Autodesk Fusion 360 part; units mm, degrees
(part 2 of 8)
  spline S29 degree 5 poles (575.857, 282.4121) (575.8643, 282.439) (575.8953, 282.5546) (575.9497, 282.7591) (576.0262, 283.0527) (576.1235, 283.4362) (576.2331, 283.8827) (576.3395, 284.3305) (576.4425, 284.7793) (576.5422, 285.2294) (576.6386, 285.6806) (576.7319, 286.1328) (576.8222, 286.5861) (576.9096, 287.0403) (576.9942, 287.4954) (577.0761, 287.9513) (577.1553, 288.4081) (577.2319, 288.8657) (577.3058, 289.3241) (577.3772, 289.7833) (577.446, 290.2433) (577.5123, 290.704) (577.5762, 291.1654) (577.6376, 291.6276) (577.6967, 292.0904) (577.7535, 292.5539) (577.8079, 293.018) (577.8601, 293.4828) (577.91, 293.9481) (577.9577, 294.4141) (578.0032, 294.8806) (578.0465, 295.3478) (578.0876, 295.8155) (578.1266, 296.2837) (578.1635, 296.7525) (578.1984, 297.2218) (578.2311, 297.6916) (578.2618, 298.1619) (578.2905, 298.6327) (578.3171, 299.1039) (578.3418, 299.5757) (578.3645, 300.0479) (578.3852, 300.5205) (578.404, 300.9936) (578.4208, 301.4672) (578.4358, 301.9411) (578.4488, 302.4154) (578.4599, 302.8902) (578.4692, 303.3654) (578.4766, 303.8409) (578.4822, 304.3168) (578.4859, 304.7931) (578.4878, 305.2698) (578.4879, 305.7468) (578.4862, 306.2242) (578.4827, 306.7019) (578.4775, 307.1799) (578.4704, 307.6583) (578.4617, 308.137) (578.4511, 308.616) (578.4389, 309.0953) (578.4249, 309.5749) (578.4123, 309.9589) (578.4021, 310.2469) (578.395, 310.4391) (578.3913, 310.5351) knots 0.13851185 0.13851185 0.13851185 0.13851185 0.13851185 0.13851185 0.14285714 0.15714286 0.17142857 0.18571429 0.2 0.21428571 0.22857143 0.24285714 0.25714286 0.27142857 0.28571429 0.3 0.31428571 0.32857143 0.34285714 0.35714286 0.37142857 0.38571429 0.4 0.41428571 0.42857143 0.44285714 0.45714286 0.47142857 0.48571429 0.5 0.51428571 0.52857143 0.54285714 0.55714286 0.57142857 0.58571429 0.6 0.61428571 0.62857143 0.64285714 0.65714286 0.67142857 0.68571429 0.7 0.71428571 0.72857143 0.74285714 0.75714286 0.77142857 0.78571429 0.8 0.81428571 0.82857143 0.84285714 0.85714286 0.87142857 0.88571429 0.9 0.91428571 0.92857143 0.94285714 0.95714286 0.97142857 0.98571429 1 1 1 1 1 1
  arc A15 (578.3913, 310.5351) -> (569.3228, 314.2914) centre (452.3696, 19.1166) ccw
  spline S30 degree 5 poles (569.3228, 314.2914) (569.2522, 314.2261) (569.1113, 314.0953) (568.9004, 313.8988) (568.62, 313.6362) (568.271, 313.307) (567.9234, 312.9767) (567.5773, 312.6455) (567.2326, 312.3132) (566.8893, 311.9799) (566.5476, 311.6456) (566.2073, 311.3103) (565.8686, 310.9739) (565.5313, 310.6365) (565.1956, 310.2982) (564.8615, 309.9587) (564.5289, 309.6183) (564.1979, 309.2768) (563.8684, 308.9342) (563.5406, 308.5906) (563.2144, 308.246) (562.8898, 307.9003) (562.5669, 307.5536) (562.2457, 307.2058) (561.9261, 306.8569) (561.6083, 306.5069) (561.2921, 306.1559) (560.9777, 305.8038) (560.6651, 305.4507) (560.3543, 305.0964) (560.0452, 304.741) (559.738, 304.3846) (559.4326, 304.027) (559.1291, 303.6683) (558.8275, 303.3085) (558.5278, 302.9476) (558.23, 302.5855) (557.9343, 302.2223) (557.6405, 301.858) (557.3488, 301.4925) (557.0591, 301.1258) (556.7715, 300.7579) (556.486, 300.3889) (556.2027, 300.0186) (555.9216, 299.6472) (555.6427, 299.2745) (555.3661, 298.9006) (555.0918, 298.5254) (554.82, 298.149) (554.5506, 297.7713) (554.2836, 297.3922) (554.0191, 297.0119) (553.7571, 296.6303) (553.4978, 296.2474) (553.2411, 295.863) (552.9873, 295.4773) (552.7364, 295.0901) (552.4887, 294.7013) (552.2441, 294.3111) (552.0027, 293.9193) (551.7645, 293.526) (551.5621, 293.1861) (551.4086, 292.9243) (551.3024, 292.7413) (551.2427, 292.6376) (551.2287, 292.6134) knots -1 -1 -1 -1 -1 -1 -0.98571429 -0.97142857 -0.95714286 -0.94285714 -0.92857143 -0.91428571 -0.9 -0.88571429 -0.87142857 -0.85714286 -0.84285714 -0.82857143 -0.81428571 -0.8 -0.78571429 -0.77142857 -0.75714286 -0.74285714 -0.72857143 -0.71428571 -0.7 -0.68571429 -0.67142857 -0.65714286 -0.64285714 -0.62857143 -0.61428571 -0.6 -0.58571429 -0.57142857 -0.55714286 -0.54285714 -0.52857143 -0.51428571 -0.5 -0.48571429 -0.47142857 -0.45714286 -0.44285714 -0.42857143 -0.41428571 -0.4 -0.38571429 -0.37142857 -0.35714286 -0.34285714 -0.32857143 -0.31428571 -0.3 -0.28571429 -0.27142857 -0.25714286 -0.24285714 -0.22857143 -0.21428571 -0.2 -0.18571429 -0.17142857 -0.15714286 -0.14285714 -0.13851185 -0.13851185 -0.13851185 -0.13851185 -0.13851185 -0.13851185
  spline S31 degree 3 poles (549.3212, 291.9095) (549.516, 291.8402) (549.7224, 291.8097) (550.1354, 291.8295) (550.338, 291.8797) (550.672, 292.0358) (550.8074, 292.1265) (551.0461, 292.3458) (551.1479, 292.473) (551.2287, 292.6134) knots 0 0 0 0 0.062015 0.062015 0.12403 0.12403 0.172638 0.172638 0.221247 0.221247 0.221247 0.221247
  arc A16 (549.3212, 291.9095) -> (541.5184, 294.5582) centre (452.3696, 19.1166) ccw
  spline S32 degree 3 poles (540.4336, 296.2779) (540.4064, 296.073) (540.4194, 295.8647) (540.5245, 295.4649) (540.6156, 295.2771) (540.8378, 294.9828) (540.9546, 294.8692) (541.2186, 294.6813) (541.3643, 294.6081) (541.5184, 294.5582) knots 0 0 0 0 0.062015 0.062015 0.12403 0.12403 0.172638 0.172638 0.221247 0.221247 0.221247 0.221247
  spline S33 degree 5 poles (540.4336, 296.2779) (540.4373, 296.3055) (540.453, 296.4242) (540.4802, 296.634) (540.5177, 296.9352) (540.5641, 297.328) (540.6146, 297.7851) (540.6615, 298.2428) (540.7051, 298.7013) (540.7452, 299.1606) (540.7819, 299.6205) (540.8153, 300.081) (540.8457, 300.5422) (540.873, 301.0039) (540.8975, 301.4661) (540.9192, 301.9288) (540.9381, 302.3921) (540.9543, 302.8557) (540.9678, 303.3199) (540.9786, 303.7845) (540.9868, 304.2495) (540.9924, 304.7149) (540.9955, 305.1808) (540.9961, 305.647) (540.9943, 306.1136) (540.9901, 306.5805) (540.9835, 307.0477) (540.9745, 307.5153) (540.9633, 307.9832) (540.9497, 308.4514) (540.9339, 308.9199) (540.9159, 309.3887) (540.8956, 309.8578) (540.8732, 310.3271) (540.8486, 310.7967) (540.8219, 311.2665) (540.793, 311.7366) (540.7621, 312.2068) (540.729, 312.6773) (540.694, 313.1481) (540.6568, 313.619) (540.6177, 314.0901) (540.5765, 314.5614) (540.5334, 315.0329) (540.4883, 315.5046) (540.4412, 315.9764) (540.3923, 316.4484) (540.3413, 316.9206) (540.2885, 317.3929) (540.2338, 317.8653) (540.1772, 318.3379) (540.1187, 318.8106) (540.0584, 319.2834) (539.9962, 319.7564) (539.9322, 320.2295) (539.8664, 320.7026) (539.7988, 321.1759) (539.7294, 321.6493) (539.6582, 322.1227) (539.5852, 322.5962) (539.5105, 323.0698) (539.434, 323.5435) (539.3715, 323.9225) (539.3237, 324.2068) (539.2916, 324.3964) (539.2754, 324.4911) knots 0.13851185 0.13851185 0.13851185 0.13851185 0.13851185 0.13851185 0.14285714 0.15714286 0.17142857 0.18571429 0.2 0.21428571 0.22857143 0.24285714 0.25714286 0.27142857 0.28571429 0.3 0.31428571 0.32857143 0.34285714 0.35714286 0.37142857 0.38571429 0.4 0.41428571 0.42857143 0.44285714 0.45714286 0.47142857 0.48571429 0.5 0.51428571 0.52857143 0.54285714 0.55714286 0.57142857 0.58571429 0.6 0.61428571 0.62857143 0.64285714 0.65714286 0.67142857 0.68571429 0.7 0.71428571 0.72857143 0.74285714 0.75714286 0.77142857 0.78571429 0.8 0.81428571 0.82857143 0.84285714 0.85714286 0.87142857 0.88571429 0.9 0.91428571 0.92857143 0.94285714 0.95714286 0.97142857 0.98571429 1 1 1 1 1 1
  arc A17 (539.2754, 324.4911) -> (529.7942, 327.0316) centre (452.3696, 19.1166) ccw
  spline S34 degree 5 poles (529.7942, 327.0316) (529.7328, 326.9576) (529.6101, 326.8096) (529.4267, 326.5872) (529.183, 326.2903) (528.8799, 325.9183) (528.5784, 325.5455) (528.2784, 325.1719) (527.9801, 324.7975) (527.6833, 324.4222) (527.3881, 324.0462) (527.0945, 323.6693) (526.8025, 323.2916) (526.5122, 322.9131) (526.2236, 322.5338) (525.9366, 322.1537) (525.6513, 321.7727) (525.3677, 321.3909) (525.0858, 321.0083) (524.8056, 320.6249) (524.5272, 320.2406) (524.2505, 319.8555) (523.9756, 319.4696) (523.7025, 319.0828) (523.4312, 318.6952) (523.1617, 318.3068) (522.8941, 317.9175) (522.6284, 317.5274) (522.3645, 317.1364) (522.1026, 316.7446) (521.8426, 316.352) (521.5845, 315.9585) (521.3284, 315.5641) (521.0743, 315.1689) (520.8222, 314.7728) (520.5722, 314.3758) (520.3243, 313.978) (520.0784, 313.5793) (519.8347, 313.1797) (519.5932, 312.7792) (519.3539, 312.3779) (519.1168, 311.9756) (518.8819, 311.5725) (518.6493, 311.1684) (518.4191, 310.7635) (518.1912, 310.3576) (517.9658, 309.9508) (517.7429, 309.543) (517.5225, 309.1343) (517.3047, 308.7246) (517.0894, 308.314) (516.8768, 307.9024) (516.6669, 307.4899) (516.4598, 307.0763) (516.2555, 306.6618) (516.0542, 306.2462) (515.856, 305.8296) (515.6611, 305.4118) (515.4696, 304.993) (515.2814, 304.5731) (515.0965, 304.152) (514.9403, 303.7886) (514.8222, 303.509) (514.7409, 303.3138) (514.6951, 303.2031) (514.6845, 303.1773) knots -1 -1 -1 -1 -1 -1 -0.98571429 -0.97142857 -0.95714286 -0.94285714 -0.92857143 -0.91428571 -0.9 -0.88571429 -0.87142857 -0.85714286 -0.84285714 -0.82857143 -0.81428571 -0.8 -0.78571429 -0.77142857 -0.75714286 -0.74285714 -0.72857143 -0.71428571 -0.7 -0.68571429 -0.67142857 -0.65714286 -0.64285714 -0.62857143 -0.61428571 -0.6 -0.58571429 -0.57142857 -0.55714286 -0.54285714 -0.52857143 -0.51428571 -0.5 -0.48571429 -0.47142857 -0.45714286 -0.44285714 -0.42857143 -0.41428571 -0.4 -0.38571429 -0.37142857 -0.35714286 -0.34285714 -0.32857143 -0.31428571 -0.3 -0.28571429 -0.27142857 -0.25714286 -0.24285714 -0.22857143 -0.21428571 -0.2 -0.18571429 -0.17142857 -0.15714286 -0.14285714 -0.13851185 -0.13851185 -0.13851185 -0.13851185 -0.13851185 -0.13851185
  spline S35 degree 3 poles (512.8852, 302.2304) (513.0873, 302.1872) (513.296, 302.1839) (513.7028, 302.2574) (513.8971, 302.3336) (514.2079, 302.532) (514.3303, 302.6396) (514.5383, 302.8881) (514.6227, 303.0276) (514.6845, 303.1773) knots 0 0 0 0 0.062015 0.062015 0.12403 0.12403 0.172638 0.172638 0.221247 0.221247 0.221247 0.221247
  arc A18 (512.8852, 302.2304) -> (504.8034, 303.838) centre (452.3696, 19.1166) ccw
  spline S36 degree 3 poles (503.5034, 305.4014) (503.5031, 305.1947) (503.5432, 304.9899) (503.6997, 304.6072) (503.8145, 304.4329) (504.0732, 304.1701) (504.2038, 304.0727) (504.4901, 303.9209) (504.644, 303.8673) (504.8034, 303.838) knots 0 0 0 0 0.062015 0.062015 0.12403 0.12403 0.172638 0.172638 0.221247 0.221247 0.221247 0.221247
  spline S37 degree 5 poles (503.5034, 305.4014) (503.5034, 305.4293) (503.5035, 305.549) (503.5031, 305.7606) (503.501, 306.064) (503.4957, 306.4596) (503.4861, 306.9193) (503.4729, 307.3793) (503.4562, 307.8395) (503.436, 308.3001) (503.4124, 308.7608) (503.3854, 309.2218) (503.3553, 309.683) (503.3222, 310.1443) (503.2861, 310.6058) (503.2472, 311.0674) (503.2055, 311.5291) (503.1611, 311.991) (503.1139, 312.4529) (503.0639, 312.9149) (503.0114, 313.377) (502.9562, 313.8392) (502.8984, 314.3015) (502.8382, 314.7638) (502.7755, 315.2261) (502.7103, 315.6885) (502.6428, 316.1509) (502.5729, 316.6133) (502.5007, 317.0757) (502.4262, 317.5382) (502.3493, 318.0006) (502.2703, 318.463) (502.1889, 318.9254) (502.1054, 319.3878) (502.0198, 319.8501) (501.9319, 320.3125) (501.842, 320.7747) (501.7499, 321.2369) (501.6557, 321.6991) (501.5595, 322.1612) (501.4612, 322.6233) (501.3609, 323.0853) (501.2586, 323.5472) (501.1543, 324.009) (501.048, 324.4708) (500.9398, 324.9324) (500.8296, 325.394) (500.7175, 325.8555) (500.6035, 326.3168) (500.4876, 326.7781) (500.3698, 327.2392) (500.2501, 327.7003) (500.1286, 328.1612) (500.0052, 328.622) (499.88, 329.0826) (499.753, 329.5431) (499.6242, 330.0035) (499.4936, 330.4638) (499.3612, 330.9239) (499.227, 331.3839) (499.0912, 331.8437) (498.9535, 332.3033) (498.842, 332.6709) (498.7576, 332.9465) (498.7009, 333.1303) (498.6725, 333.2221) knots 0.13851185 0.13851185 0.13851185 0.13851185 0.13851185 0.13851185 0.14285714 0.15714286 0.17142857 0.18571429 0.2 0.21428571 0.22857143 0.24285714 0.25714286 0.27142857 0.28571429 0.3 0.31428571 0.32857143 0.34285714 0.35714286 0.37142857 0.38571429 0.4 0.41428571 0.42857143 0.44285714 0.45714286 0.47142857 0.48571429 0.5 0.51428571 0.52857143 0.54285714 0.55714286 0.57142857 0.58571429 0.6 0.61428571 0.62857143 0.64285714 0.65714286 0.67142857 0.68571429 0.7 0.71428571 0.72857143 0.74285714 0.75714286 0.77142857 0.78571429 0.8 0.81428571 0.82857143 0.84285714 0.85714286 0.87142857 0.88571429 0.9 0.91428571 0.92857143 0.94285714 0.95714286 0.97142857 0.98571429 1 1 1 1 1 1
  arc A19 (498.6725, 333.2221) -> (488.9408, 334.5033) centre (452.3696, 19.1166) ccw
  spline S38 degree 5 poles (488.9408, 334.5033) (488.8896, 334.422) (488.7873, 334.2591) (488.6345, 334.0148) (488.4316, 333.6885) (488.1797, 333.2802) (487.9294, 332.8712) (487.6808, 332.4617) (487.4338, 332.0515) (487.1886, 331.6407) (486.945, 331.2294) (486.7031, 330.8174) (486.4629, 330.4048) (486.2245, 329.9917) (485.9878, 329.5779) (485.7529, 329.1636) (485.5198, 328.7486) (485.2884, 328.3331) (485.0589, 327.9169) (484.8312, 327.5002) (484.6053, 327.0829) (484.3812, 326.665) (484.1591, 326.2465) (483.9388, 325.8274) (483.7204, 325.4077) (483.5039, 324.9874) (483.2894, 324.5665) (483.0769, 324.1451) (482.8663, 323.723) (482.6577, 323.3004) (482.4512, 322.8771) (482.2467, 322.4533) (482.0443, 322.0289) (481.8439, 321.6039) (481.6457, 321.1783) (481.4497, 320.7521) (481.2558, 320.3253) (481.0641, 319.8979) (480.8746, 319.4699) (480.6874, 319.0414) (480.5025, 318.6122) (480.3199, 318.1824) (480.1397, 317.7521) (479.9619, 317.3211) (479.7864, 316.8896) (479.6135, 316.4574) (479.4431, 316.0247) (479.2753, 315.5913) (479.1102, 315.1573) (478.9477, 314.7227) (478.7879, 314.2875) (478.6309, 313.8517) (478.4766, 313.4153) (478.3252, 312.9783) (478.1767, 312.5406) (478.0314, 312.1023) (477.8893, 311.6634) (477.7506, 311.2238) (477.6154, 310.7835) (477.4836, 310.3426) (477.3553, 309.901) (477.2478, 309.5203) (477.1673, 309.2277) (477.1121, 309.0235) (477.0812, 308.9079) (477.074, 308.8809) knots -1 -1 -1 -1 -1 -1 -0.98571429 -0.97142857 -0.95714286 -0.94285714 -0.92857143 -0.91428571 -0.9 -0.88571429 -0.87142857 -0.85714286 -0.84285714 -0.82857143 -0.81428571 -0.8 -0.78571429 -0.77142857 -0.75714286 -0.74285714 -0.72857143 -0.71428571 -0.7 -0.68571429 -0.67142857 -0.65714286 -0.64285714 -0.62857143 -0.61428571 -0.6 -0.58571429 -0.57142857 -0.55714286 -0.54285714 -0.52857143 -0.51428571 -0.5 -0.48571429 -0.47142857 -0.45714286 -0.44285714 -0.42857143 -0.41428571 -0.4 -0.38571429 -0.37142857 -0.35714286 -0.34285714 -0.32857143 -0.31428571 -0.3 -0.28571429 -0.27142857 -0.25714286 -0.24285714 -0.22857143 -0.21428571 -0.2 -0.18571429 -0.17142857 -0.15714286 -0.14285714 -0.13851185 -0.13851185 -0.13851185 -0.13851185 -0.13851185 -0.13851185
  spline S39 degree 3 poles (475.4137, 307.7072) (475.6197, 307.6908) (475.827, 307.7147) (476.2208, 307.8407) (476.4035, 307.9416) (476.6857, 308.1789) (476.793, 308.3015) (476.9668, 308.5751) (477.0323, 308.7243) (477.074, 308.8809) knots 0 0 0 0 0.062015 0.062015 0.12403 0.12403 0.172638 0.172638 0.221247 0.221247 0.221247 0.221247
  arc A20 (475.4137, 307.7072) -> (467.1912, 308.2461) centre (452.3696, 19.1166) ccw
  spline S40 degree 3 poles (465.6983, 309.6265) (465.725, 309.4215) (465.7915, 309.2237) (465.9965, 308.8647) (466.1331, 308.7069) (466.4239, 308.4802) (466.5662, 308.4006) (466.8698, 308.2875) (467.0294, 308.2544) (467.1912, 308.2461) knots 0 0 0 0 0.062015 0.062015 0.12403 0.12403 0.172638 0.172638 0.221247 0.221247 0.221247 0.221247
  spline S41 degree 5 poles (465.6983, 309.6265) (465.6947, 309.6542) (465.6791, 309.7729) (465.6511, 309.9825) (465.6094, 310.2831) (465.5526, 310.6746) (465.483, 311.1291) (465.4099, 311.5835) (465.3333, 312.0376) (465.2531, 312.4916) (465.1695, 312.9453) (465.0827, 313.3988) (464.9926, 313.8521) (464.8996, 314.3052) (464.8036, 314.758) (464.7048, 315.2106) (464.6031, 315.6629) (464.4988, 316.115) (464.3917, 316.5668) (464.2819, 317.0184) (464.1694, 317.4697) (464.0544, 317.9207) (463.9368, 318.3715) (463.8167, 318.8219) (463.6942, 319.2721) (463.5693, 319.7221) (463.442, 320.1717) (463.3123, 320.621) (463.1803, 321.0701) (463.0461, 321.5188) (462.9096, 321.9673) (462.7708, 322.4154) (462.6298, 322.8632) (462.4867, 323.3108) (462.3414, 323.758) (462.194, 324.2049) (462.0444, 324.6514) (461.8928, 325.0977) (461.7391, 325.5436) (461.5834, 325.9892) (461.4257, 326.4345) (461.2659, 326.8794) (461.1042, 327.324) (460.9405, 327.7683) (460.7749, 328.2122) (460.6073, 328.6558) (460.4378, 329.099) (460.2664, 329.5419) (460.0932, 329.9845) (459.918, 330.4266) (459.741, 330.8685) (459.5622, 331.3099) (459.3816, 331.751) (459.1991, 332.1918) (459.0149, 332.6322) (458.8288, 333.0722) (458.641, 333.5118) (458.4515, 333.9511) (458.2601, 334.39) (458.0671, 334.8285) (457.8724, 335.2666) (457.6759, 335.7044) (457.5174, 336.0543) (457.3977, 336.3165) (457.3176, 336.4913) (457.2774, 336.5787) knots 0.13851185 0.13851185 0.13851185 0.13851185 0.13851185 0.13851185 0.14285714 0.15714286 0.17142857 0.18571429 0.2 0.21428571 0.22857143 0.24285714 0.25714286 0.27142857 0.28571429 0.3 0.31428571 0.32857143 0.34285714 0.35714286 0.37142857 0.38571429 0.4 0.41428571 0.42857143 0.44285714 0.45714286 0.47142857 0.48571429 0.5 0.51428571 0.52857143 0.54285714 0.55714286 0.57142857 0.58571429 0.6 0.61428571 0.62857143 0.64285714 0.65714286 0.67142857 0.68571429 0.7 0.71428571 0.72857143 0.74285714 0.75714286 0.77142857 0.78571429 0.8 0.81428571 0.82857143 0.84285714 0.85714286 0.87142857 0.88571429 0.9 0.91428571 0.92857143 0.94285714 0.95714286 0.97142857 0.98571429 1 1 1 1 1 1
  arc A21 (457.2774, 336.5787) -> (447.4617, 336.5787) centre (452.3696, 19.1166) ccw
  spline S42 degree 5 poles (447.4617, 336.5787) (447.4215, 336.4913) (447.3414, 336.3165) (447.2217, 336.0543) (447.0632, 335.7044) (446.8667, 335.2666) (446.672, 334.8285) (446.479, 334.39) (446.2877, 333.9511) (446.0981, 333.5118) (445.9103, 333.0722) (445.7242, 332.6322) (445.54, 332.1918) (445.3575, 331.751) (445.1769, 331.3099) (444.9981, 330.8685) (444.8211, 330.4266) (444.6459, 329.9845) (444.4727, 329.5419) (444.3013, 329.099) (444.1318, 328.6558) (443.9642, 328.2122) (443.7986, 327.7683) (443.6349, 327.324) (443.4732, 326.8794) (443.3134, 326.4345) (443.1557, 325.9892) (443, 325.5436) (442.8463, 325.0977) (442.6947, 324.6514) (442.5451, 324.2049) (442.3977, 323.758) (442.2524, 323.3108) (442.1093, 322.8632) (441.9683, 322.4154) (441.8295, 321.9673) (441.693, 321.5188) (441.5588, 321.0701) (441.4268, 320.621) (441.2971, 320.1717) (441.1698, 319.7221) (441.0449, 319.2721) (440.9224, 318.8219) (440.8023, 318.3715) (440.6847, 317.9207) (440.5697, 317.4697) (440.4572, 317.0184) (440.3474, 316.5668) (440.2403, 316.115) (440.136, 315.6629) (440.0344, 315.2106) (439.9355, 314.758) (439.8395, 314.3052) (439.7465, 313.8521) (439.6564, 313.3988) (439.5696, 312.9453) (439.486, 312.4916) (439.4059, 312.0376) (439.3292, 311.5835) (439.2561, 311.1291) (439.1866, 310.6746) (439.1297, 310.2831) (439.088, 309.9825) (439.06, 309.7729) (439.0444, 309.6542) (439.0408, 309.6265) knots -1 -1 -1 -1 -1 -1 -0.98571429 -0.97142857 -0.95714286 -0.94285714 -0.92857143 -0.91428571 -0.9 -0.88571429 -0.87142857 -0.85714286 -0.84285714 -0.82857143 -0.81428571 -0.8 -0.78571429 -0.77142857 -0.75714286 -0.74285714 -0.72857143 -0.71428571 -0.7 -0.68571429 -0.67142857 -0.65714286 -0.64285714 -0.62857143 -0.61428571 -0.6 -0.58571429 -0.57142857 -0.55714286 -0.54285714 -0.52857143 -0.51428571 -0.5 -0.48571429 -0.47142857 -0.45714286 -0.44285714 -0.42857143 -0.41428571 -0.4 -0.38571429 -0.37142857 -0.35714286 -0.34285714 -0.32857143 -0.31428571 -0.3 -0.28571429 -0.27142857 -0.25714286 -0.24285714 -0.22857143 -0.21428571 -0.2 -0.18571429 -0.17142857 -0.15714286 -0.14285714 -0.13851185 -0.13851185 -0.13851185 -0.13851185 -0.13851185 -0.13851185
  spline S43 degree 3 poles (437.5479, 308.2461) (437.7543, 308.2567) (437.9567, 308.3075) (438.3307, 308.4839) (438.4986, 308.6077) (438.7475, 308.8798) (438.8379, 309.0154) (438.9745, 309.3093) (439.0199, 309.4658) (439.0408, 309.6265) knots 0 0 0 0 0.062015 0.062015 0.12403 0.12403 0.172638 0.172638 0.221247 0.221247 0.221247 0.221247
  arc A22 (437.5479, 308.2461) -> (429.3254, 307.7072) centre (452.3696, 19.1166) ccw
  spline S44 degree 3 poles (427.6651, 308.8809) (427.7183, 308.6811) (427.8101, 308.4937) (428.0602, 308.1645) (428.2163, 308.026) (428.5341, 307.8391) (428.6856, 307.7788) (429.0014, 307.7062) (429.1639, 307.6943) (429.3254, 307.7072) knots 0 0 0 0 0.062015 0.062015 0.12403 0.12403 0.172638 0.172638 0.221247 0.221247 0.221247 0.221247
  spline S45 degree 5 poles (427.6651, 308.8809) (427.6579, 308.9079) (427.627, 309.0235) (427.5718, 309.2277) (427.4913, 309.5203) (427.3838, 309.901) (427.2555, 310.3426) (427.1237, 310.7835) (426.9885, 311.2238) (426.8498, 311.6634) (426.7077, 312.1023) (426.5624, 312.5406) (426.4139, 312.9783) (426.2625, 313.4153) (426.1082, 313.8517) (425.9512, 314.2875) (425.7914, 314.7227) (425.6289, 315.1573) (425.4638, 315.5913) (425.296, 316.0247) (425.1256, 316.4574) (424.9527, 316.8896) (424.7772, 317.3211) (424.5994, 317.7521) (424.4192, 318.1824) (424.2366, 318.6122) (424.0517, 319.0414) (423.8645, 319.4699) (423.675, 319.8979) (423.4833, 320.3253) (423.2894, 320.7521) (423.0934, 321.1783) (422.8952, 321.6039) (422.6948, 322.0289) (422.4924, 322.4533) (422.2879, 322.8771) (422.0814, 323.3004) (421.8728, 323.723) (421.6622, 324.1451) (421.4497, 324.5665) (421.2352, 324.9874) (421.0187, 325.4077) (420.8003, 325.8274) (420.5801, 326.2465) (420.3579, 326.665) (420.1338, 327.0829) (419.908, 327.5002) (419.6802, 327.9169) (419.4507, 328.3331) (419.2193, 328.7486) (418.9862, 329.1636) (418.7513, 329.5779) (418.5146, 329.9917) (418.2762, 330.4048) (418.036, 330.8174) (417.7941, 331.2294) (417.5505, 331.6407) (417.3053, 332.0515) (417.0583, 332.4617) (416.8097, 332.8712) (416.5594, 333.2802) (416.3075, 333.6885) (416.1046, 334.0148) (415.9518, 334.2591) (415.8495, 334.422) (415.7983, 334.5033) knots 0.13851185 0.13851185 0.13851185 0.13851185 0.13851185 0.13851185 0.14285714 0.15714286 0.17142857 0.18571429 0.2 0.21428571 0.22857143 0.24285714 0.25714286 0.27142857 0.28571429 0.3 0.31428571 0.32857143 0.34285714 0.35714286 0.37142857 0.38571429 0.4 0.41428571 0.42857143 0.44285714 0.45714286 0.47142857 0.48571429 0.5 0.51428571 0.52857143 0.54285714 0.55714286 0.57142857 0.58571429 0.6 0.61428571 0.62857143 0.64285714 0.65714286 0.67142857 0.68571429 0.7 0.71428571 0.72857143 0.74285714 0.75714286 0.77142857 0.78571429 0.8 0.81428571 0.82857143 0.84285714 0.85714286 0.87142857 0.88571429 0.9 0.91428571 0.92857143 0.94285714 0.95714286 0.97142857 0.98571429 1 1 1 1 1 1
  arc A23 (415.7983, 334.5033) -> (406.0666, 333.2221) centre (452.3696, 19.1166) ccw
  spline S46 degree 5 poles (406.0666, 333.2221) (406.0382, 333.1303) (405.9815, 332.9465) (405.8971, 332.6709) (405.7856, 332.3033) (405.648, 331.8437) (405.5121, 331.3839) (405.3779, 330.9239) (405.2455, 330.4638) (405.1149, 330.0035) (404.9861, 329.5431) (404.8591, 329.0826) (404.7339, 328.622) (404.6105, 328.1612) (404.489, 327.7003) (404.3693, 327.2392) (404.2515, 326.7781) (404.1356, 326.3168) (404.0216, 325.8555) (403.9095, 325.394) (403.7993, 324.9324) (403.6911, 324.4708) (403.5848, 324.009) (403.4805, 323.5472) (403.3782, 323.0853) (403.2779, 322.6233) (403.1796, 322.1612) (403.0834, 321.6991) (402.9892, 321.2369) (402.8971, 320.7747) (402.8072, 320.3125) (402.7194, 319.8501) (402.6337, 319.3878) (402.5502, 318.9254) (402.4689, 318.463) (402.3898, 318.0006) (402.3129, 317.5382) (402.2384, 317.0757) (402.1662, 316.6133) (402.0963, 316.1509) (402.0288, 315.6885) (401.9636, 315.2261) (401.9009, 314.7638) (401.8407, 314.3015) (401.7829, 313.8392) (401.7277, 313.377) (401.6752, 312.9149) (401.6252, 312.4529) (401.578, 311.991) (401.5336, 311.5291) (401.4919, 311.0674) (401.453, 310.6058) (401.4169, 310.1443) (401.3838, 309.683) (401.3537, 309.2218) (401.3267, 308.7608) (401.3031, 308.3001) (401.2829, 307.8395) (401.2662, 307.3793) (401.253, 306.9193) (401.2434, 306.4596) (401.2381, 306.064) (401.236, 305.7606) (401.2356, 305.549) (401.2357, 305.4293) (401.2357, 305.4014) knots -1 -1 -1 -1 -1 -1 -0.98571429 -0.97142857 -0.95714286 -0.94285714 -0.92857143 -0.91428571 -0.9 -0.88571429 -0.87142857 -0.85714286 -0.84285714 -0.82857143 -0.81428571 -0.8 -0.78571429 -0.77142857 -0.75714286 -0.74285714 -0.72857143 -0.71428571 -0.7 -0.68571429 -0.67142857 -0.65714286 -0.64285714 -0.62857143 -0.61428571 -0.6 -0.58571429 -0.57142857 -0.55714286 -0.54285714 -0.52857143 -0.51428571 -0.5 -0.48571429 -0.47142857 -0.45714286 -0.44285714 -0.42857143 -0.41428571 -0.4 -0.38571429 -0.37142857 -0.35714286 -0.34285714 -0.32857143 -0.31428571 -0.3 -0.28571429 -0.27142857 -0.25714286 -0.24285714 -0.22857143 -0.21428571 -0.2 -0.18571429 -0.17142857 -0.15714286 -0.14285714 -0.13851185 -0.13851185 -0.13851185 -0.13851185 -0.13851185 -0.13851185
  spline S47 degree 3 poles (399.9357, 303.838) (400.139, 303.8754) (400.3331, 303.9522) (400.6808, 304.1758) (400.8311, 304.3205) (401.0423, 304.6228) (401.1143, 304.7691) (401.2113, 305.0782) (401.2359, 305.2394) (401.2357, 305.4014) knots 0 0 0 0 0.062015 0.062015 0.12403 0.12403 0.172638 0.172638 0.221247 0.221247 0.221247 0.221247
  arc A24 (399.9357, 303.838) -> (391.8539, 302.2304) centre (452.3696, 19.1166) ccw
  spline S48 degree 3 poles (390.0546, 303.1773) (390.1335, 302.9862) (390.2489, 302.8124) (390.5399, 302.5187) (390.7126, 302.4017) (391.0522, 302.2579) (391.2102, 302.2179) (391.5328, 302.1871) (391.6955, 302.1965) (391.8539, 302.2304) knots 0 0 0 0 0.062015 0.062015 0.12403 0.12403 0.172638 0.172638 0.221247 0.221247 0.221247 0.221247
  spline S49 degree 5 poles (390.0546, 303.1773) (390.044, 303.2031) (389.9982, 303.3138) (389.9169, 303.509) (389.7988, 303.7886) (389.6426, 304.152) (389.4577, 304.5731) (389.2695, 304.993) (389.078, 305.4118) (388.8831, 305.8296) (388.6849, 306.2462) (388.4836, 306.6618) (388.2793, 307.0763) (388.0722, 307.4899) (387.8623, 307.9024) (387.6497, 308.314) (387.4344, 308.7246) (387.2166, 309.1343) (386.9962, 309.543) (386.7733, 309.9508) (386.5479, 310.3576) (386.32, 310.7635) (386.0898, 311.1684) (385.8572, 311.5725) (385.6224, 311.9756) (385.3852, 312.3779) (385.1459, 312.7792) (384.9044, 313.1797) (384.6607, 313.5793) (384.4148, 313.978) (384.1669, 314.3758) (383.9169, 314.7728) (383.6648, 315.1689) (383.4107, 315.5641) (383.1546, 315.9585) (382.8965, 316.352) (382.6365, 316.7446) (382.3746, 317.1364) (382.1107, 317.5274) (381.845, 317.9175) (381.5774, 318.3068) (381.3079, 318.6952) (381.0366, 319.0828) (380.7635, 319.4696) (380.4886, 319.8555) (380.212, 320.2406) (379.9335, 320.6249) (379.6534, 321.0083) (379.3715, 321.3909) (379.0878, 321.7727) (378.8025, 322.1537) (378.5155, 322.5338) (378.2269, 322.9131) (377.9366, 323.2916) (377.6446, 323.6693) (377.351, 324.0462) (377.0558, 324.4222) (376.759, 324.7975) (376.4607, 325.1719) (376.1607, 325.5455) (375.8592, 325.9183) (375.5561, 326.2903) (375.3124, 326.5872) (375.129, 326.8096) (375.0063, 326.9576) (374.945, 327.0316) knots 0.13851185 0.13851185 0.13851185 0.13851185 0.13851185 0.13851185 0.14285714 0.15714286 0.17142857 0.18571429 0.2 0.21428571 0.22857143 0.24285714 0.25714286 0.27142857 0.28571429 0.3 0.31428571 0.32857143 0.34285714 0.35714286 0.37142857 0.38571429 0.4 0.41428571 0.42857143 0.44285714 0.45714286 0.47142857 0.48571429 0.5 0.51428571 0.52857143 0.54285714 0.55714286 0.57142857 0.58571429 0.6 0.61428571 0.62857143 0.64285714 0.65714286 0.67142857 0.68571429 0.7 0.71428571 0.72857143 0.74285714 0.75714286 0.77142857 0.78571429 0.8 0.81428571 0.82857143 0.84285714 0.85714286 0.87142857 0.88571429 0.9 0.91428571 0.92857143 0.94285714 0.95714286 0.97142857 0.98571429 1 1 1 1 1 1
  arc A25 (374.945, 327.0316) -> (365.4637, 324.4911) centre (452.3696, 19.1166) ccw
  spline S50 degree 5 poles (365.4637, 324.4911) (365.4475, 324.3964) (365.4154, 324.2068) (365.3676, 323.9225) (365.3051, 323.5435) (365.2286, 323.0698) (365.1539, 322.5962) (365.0809, 322.1227) (365.0097, 321.6493) (364.9403, 321.1759) (364.8727, 320.7026) (364.8069, 320.2295) (364.7429, 319.7564) (364.6807, 319.2834) (364.6204, 318.8106) (364.5619, 318.3379) (364.5053, 317.8653) (364.4506, 317.3929) (364.3978, 316.9206) (364.3469, 316.4484) (364.2979, 315.9764) (364.2508, 315.5046) (364.2057, 315.0329) (364.1626, 314.5614) (364.1214, 314.0901) (364.0823, 313.619) (364.0452, 313.1481) (364.0101, 312.6773) (363.977, 312.2068) (363.9461, 311.7366) (363.9172, 311.2665) (363.8905, 310.7967) (363.8659, 310.3271) (363.8435, 309.8578) (363.8232, 309.3887) (363.8052, 308.9199) (363.7894, 308.4514) (363.7758, 307.9832) (363.7646, 307.5153) (363.7556, 307.0477) (363.749, 306.5805) (363.7448, 306.1136) (363.743, 305.647) (363.7436, 305.1808) (363.7467, 304.7149) (363.7523, 304.2495) (363.7605, 303.7845) (363.7713, 303.3199) (363.7848, 302.8557) (363.801, 302.3921) (363.8199, 301.9288) (363.8416, 301.4661) (363.8661, 301.0039) (363.8934, 300.5422) (363.9238, 300.081) (363.9572, 299.6205) (363.994, 299.1606) (364.034, 298.7013) (364.0776, 298.2428) (364.1246, 297.7851) (364.175, 297.328) (364.2214, 296.9352) (364.2589, 296.634) (364.2861, 296.4242) (364.3018, 296.3055) (364.3055, 296.2779) knots -1 -1 -1 -1 -1 -1 -0.98571429 -0.97142857 -0.95714286 -0.94285714 -0.92857143 -0.91428571 -0.9 -0.88571429 -0.87142857 -0.85714286 -0.84285714 -0.82857143 -0.81428571 -0.8 -0.78571429 -0.77142857 -0.75714286 -0.74285714 -0.72857143 -0.71428571 -0.7 -0.68571429 -0.67142857 -0.65714286 -0.64285714 -0.62857143 -0.61428571 -0.6 -0.58571429 -0.57142857 -0.55714286 -0.54285714 -0.52857143 -0.51428571 -0.5 -0.48571429 -0.47142857 -0.45714286 -0.44285714 -0.42857143 -0.41428571 -0.4 -0.38571429 -0.37142857 -0.35714286 -0.34285714 -0.32857143 -0.31428571 -0.3 -0.28571429 -0.27142857 -0.25714286 -0.24285714 -0.22857143 -0.21428571 -0.2 -0.18571429 -0.17142857 -0.15714286 -0.14285714 -0.13851185 -0.13851185 -0.13851185 -0.13851185 -0.13851185 -0.13851185
  spline S51 degree 3 poles (363.2207, 294.5582) (363.4174, 294.6218) (363.5997, 294.7233) (363.9153, 294.9904) (364.0455, 295.1535) (364.2154, 295.4807) (364.2676, 295.6351) (364.3235, 295.9543) (364.3269, 296.1173) (364.3055, 296.2779) knots 0 0 0 0 0.062015 0.062015 0.12403 0.12403 0.172638 0.172638 0.221247 0.221247 0.221247 0.221247
  arc A26 (363.2207, 294.5582) -> (355.4179, 291.9095) centre (452.3696, 19.1166) ccw
  spline S52 degree 3 poles (353.5104, 292.6134) (353.6135, 292.4343) (353.7506, 292.277) (354.0774, 292.0238) (354.264, 291.9303) (354.6194, 291.832) (354.7813, 291.813) (355.1051, 291.8246) (355.2652, 291.8552) (355.4179, 291.9095) knots 0 0 0 0 0.062015 0.062015 0.12403 0.12403 0.172638 0.172638 0.221247 0.221247 0.221247 0.221247
  spline S53 degree 5 poles (353.5104, 292.6134) (353.4964, 292.6376) (353.4367, 292.7413) (353.3305, 292.9243) (353.177, 293.1861) (352.9746, 293.526) (352.7364, 293.9193) (352.495, 294.3111) (352.2504, 294.7013) (352.0027, 295.0901) (351.7518, 295.4773) (351.498, 295.863) (351.2413, 296.2474) (350.982, 296.6303) (350.72, 297.0119) (350.4555, 297.3922) (350.1885, 297.7713) (349.9191, 298.149) (349.6473, 298.5254) (349.373, 298.9006) (349.0964, 299.2745) (348.8175, 299.6472) (348.5364, 300.0186) (348.2531, 300.3889) (347.9676, 300.7579) (347.68, 301.1258) (347.3903, 301.4925) (347.0986, 301.858) (346.8048, 302.2223) (346.5091, 302.5855) (346.2113, 302.9476) (345.9116, 303.3085) (345.61, 303.6683) (345.3065, 304.027) (345.0011, 304.3846) (344.6939, 304.741) (344.3848, 305.0964) (344.074, 305.4507) (343.7614, 305.8038) (343.447, 306.1559) (343.1309, 306.5069) (342.813, 306.8569) (342.4934, 307.2058) (342.1722, 307.5536) (341.8493, 307.9003) (341.5247, 308.246) (341.1985, 308.5906) (340.8707, 308.9342) (340.5412, 309.2768) (340.2102, 309.6183) (339.8776, 309.9587) (339.5435, 310.2982) (339.2078, 310.6365) (338.8705, 310.9739) (338.5318, 311.3103) (338.1915, 311.6456) (337.8498, 311.9799) (337.5065, 312.3132) (337.1618, 312.6455) (336.8157, 312.9767) (336.4681, 313.307) (336.1191, 313.6362) (335.8387, 313.8988) (335.6278, 314.0953) (335.4869, 314.2261) (335.4164, 314.2914) knots 0.13851185 0.13851185 0.13851185 0.13851185 0.13851185 0.13851185 0.14285714 0.15714286 0.17142857 0.18571429 0.2 0.21428571 0.22857143 0.24285714 0.25714286 0.27142857 0.28571429 0.3 0.31428571 0.32857143 0.34285714 0.35714286 0.37142857 0.38571429 0.4 0.41428571 0.42857143 0.44285714 0.45714286 0.47142857 0.48571429 0.5 0.51428571 0.52857143 0.54285714 0.55714286 0.57142857 0.58571429 0.6 0.61428571 0.62857143 0.64285714 0.65714286 0.67142857 0.68571429 0.7 0.71428571 0.72857143 0.74285714 0.75714286 0.77142857 0.78571429 0.8 0.81428571 0.82857143 0.84285714 0.85714286 0.87142857 0.88571429 0.9 0.91428571 0.92857143 0.94285714 0.95714286 0.97142857 0.98571429 1 1 1 1 1 1
  arc A27 (335.4164, 314.2914) -> (326.3478, 310.5351) centre (452.3696, 19.1166) ccw
  spline S54 degree 5 poles (326.3478, 310.5351) (326.3441, 310.4391) (326.337, 310.2469) (326.3268, 309.9589) (326.3142, 309.5749) (326.3002, 309.0953) (326.288, 308.616) (326.2774, 308.137) (326.2687, 307.6583) (326.2616, 307.1799) (326.2564, 306.7019) (326.2529, 306.2242) (326.2512, 305.7468) (326.2513, 305.2698) (326.2532, 304.7931) (326.2569, 304.3168) (326.2625, 303.8409) (326.2699, 303.3654) (326.2792, 302.8902) (326.2903, 302.4154) (326.3033, 301.9411) (326.3183, 301.4672) (326.3351, 300.9936) (326.3539, 300.5205) (326.3746, 300.0479) (326.3973, 299.5757) (326.422, 299.1039) (326.4486, 298.6327) (326.4773, 298.1619) (326.508, 297.6916) (326.5408, 297.2218) (326.5756, 296.7525) (326.6125, 296.2837) (326.6515, 295.8155) (326.6926, 295.3478) (326.7359, 294.8806) (326.7814, 294.4141) (326.8291, 293.9481) (326.879, 293.4828) (326.9312, 293.018) (326.9856, 292.5539) (327.0424, 292.0904) (327.1015, 291.6276) (327.1629, 291.1654) (327.2268, 290.704) (327.2931, 290.2433) (327.3619, 289.7833) (327.4333, 289.3241) (327.5073, 288.8657) (327.5838, 288.4081) (327.663, 287.9513) (327.7449, 287.4954) (327.8296, 287.0403) (327.9169, 286.5861) (328.0072, 286.1328) (328.1005, 285.6806) (328.1969, 285.2294) (328.2966, 284.7793) (328.3996, 284.3305) (328.506, 283.8827) (328.6156, 283.4362) (328.7129, 283.0527) (328.7894, 282.7591) (328.8438, 282.5546) (328.8748, 282.439) (328.8821, 282.4121) knots -1 -1 -1 -1 -1 -1 -0.98571429 -0.97142857 -0.95714286 -0.94285714 -0.92857143 -0.91428571 -0.9 -0.88571429 -0.87142857 -0.85714286 -0.84285714 -0.82857143 -0.81428571 -0.8 -0.78571429 -0.77142857 -0.75714286 -0.74285714 -0.72857143 -0.71428571 -0.7 -0.68571429 -0.67142857 -0.65714286 -0.64285714 -0.62857143 -0.61428571 -0.6 -0.58571429 -0.57142857 -0.55714286 -0.54285714 -0.52857143 -0.51428571 -0.5 -0.48571429 -0.47142857 -0.45714286 -0.44285714 -0.42857143 -0.41428571 -0.4 -0.38571429 -0.37142857 -0.35714286 -0.34285714 -0.32857143 -0.31428571 -0.3 -0.28571429 -0.27142857 -0.25714286 -0.24285714 -0.22857143 -0.21428571 -0.2 -0.18571429 -0.17142857 -0.15714286 -0.14285714 -0.13851185 -0.13851185 -0.13851185 -0.13851185 -0.13851185 -0.13851185
  spline S55 degree 3 poles (328.031, 280.5655) (328.2177, 280.6542) (328.3853, 280.7786) (328.6633, 281.0846) (328.7711, 281.2633) (328.8968, 281.61) (328.9284, 281.7699) (328.9422, 282.0936) (328.9242, 282.2556) (328.8821, 282.4121) knots 0 0 0 0 0.062015 0.062015 0.12403 0.12403 0.172638 0.172638 0.221247 0.221247 0.221247 0.221247
  arc A28 (328.031, 280.5655) -> (320.6407, 276.9209) centre (452.3696, 19.1166) ccw
  spline S56 degree 3 poles (318.6576, 277.3699) (318.7832, 277.2057) (318.9397, 277.0677) (319.2968, 276.8593) (319.494, 276.791) (319.8592, 276.7399) (320.0221, 276.7422) (320.3417, 276.796) (320.4964, 276.8472) (320.6407, 276.9209) knots 0 0 0 0 0.062015 0.062015 0.12403 0.12403 0.172638 0.172638 0.221247 0.221247 0.221247 0.221247
  spline S57 degree 5 poles (318.6576, 277.3699) (318.6407, 277.3921) (318.5679, 277.4871) (318.4387, 277.6547) (318.2523, 277.8942) (318.0074, 278.2047) (317.7198, 278.5636) (317.4294, 278.9205) (317.1359, 279.2755) (316.8396, 279.6286) (316.5403, 279.9797) (316.2383, 280.329) (315.9337, 280.6766) (315.6266, 281.0224) (315.317, 281.3666) (315.0051, 281.7091) (314.691, 282.05) (314.3746, 282.3894) (314.0559, 282.7271) (313.735, 283.0633) (313.412, 283.3979) (313.0869, 283.731) (312.7596, 284.0625) (312.4304, 284.3926) (312.0992, 284.7213) (311.7661, 285.0484) (311.431, 285.3742) (311.094, 285.6985) (310.7552, 286.0214) (310.4146, 286.3429) (310.0721, 286.663) (309.7279, 286.9817) (309.3819, 287.299) (309.0342, 287.615) (308.6847, 287.9297) (308.3336, 288.243) (307.9808, 288.555) (307.6264, 288.8656) (307.2703, 289.175) (306.9127, 289.483) (306.5534, 289.7898) (306.1926, 290.0952) (305.8303, 290.3994) (305.4664, 290.7023) (305.1009, 291.0039) (304.734, 291.3043) (304.3656, 291.6034) (303.9958, 291.9013) (303.6245, 292.1979) (303.2517, 292.4932) (302.8775, 292.7874) (302.5019, 293.0803) (302.1249, 293.372) (301.7465, 293.6624) (301.3668, 293.9517) (300.9856, 294.2397) (300.6032, 294.5266) (300.2194, 294.8122) (299.8343, 295.0967) (299.4478, 295.3799) (299.0601, 295.662) (298.6711, 295.9428) (298.3588, 296.1666) (298.1241, 296.3339) (297.9673, 296.4451) (297.8889, 296.5007) knots 0.13851185 0.13851185 0.13851185 0.13851185 0.13851185 0.13851185 0.14285714 0.15714286 0.17142857 0.18571429 0.2 0.21428571 0.22857143 0.24285714 0.25714286 0.27142857 0.28571429 0.3 0.31428571 0.32857143 0.34285714 0.35714286 0.37142857 0.38571429 0.4 0.41428571 0.42857143 0.44285714 0.45714286 0.47142857 0.48571429 0.5 0.51428571 0.52857143 0.54285714 0.55714286 0.57142857 0.58571429 0.6 0.61428571 0.62857143 0.64285714 0.65714286 0.67142857 0.68571429 0.7 0.71428571 0.72857143 0.74285714 0.75714286 0.77142857 0.78571429 0.8 0.81428571 0.82857143 0.84285714 0.85714286 0.87142857 0.88571429 0.9 0.91428571 0.92857143 0.94285714 0.95714286 0.97142857 0.98571429 1 1 1 1 1 1
  arc A29 (297.8889, 296.5007) -> (289.3882, 291.5929) centre (452.3696, 19.1166) ccw
  spline S58 degree 5 poles (289.3882, 291.5929) (289.3971, 291.4971) (289.4151, 291.3057) (289.4426, 291.0188) (289.4802, 290.6365) (289.529, 290.1591) (289.5794, 289.6823) (289.6314, 289.2061) (289.6852, 288.7303) (289.7407, 288.2551) (289.7979, 287.7805) (289.8568, 287.3064) (289.9174, 286.8329) (289.9797, 286.36) (290.0438, 285.8876) (290.1097, 285.4159) (290.1774, 284.9448) (290.2468, 284.4743) (290.318, 284.0044) (290.391, 283.5351) (290.4658, 283.0665) (290.5425, 282.5986) (290.621, 282.1313) (290.7014, 281.6647) (290.7836, 281.1988) (290.8678, 280.7336) (290.9538, 280.2692) (291.0417, 279.8054) (291.1316, 279.3424) (291.2234, 278.8801) (291.3172, 278.4186) (291.413, 277.9578) (291.5108, 277.4979) (291.6106, 277.0388) (291.7124, 276.5804) (291.8163, 276.123) (291.9223, 275.6663) (292.0304, 275.2106) (292.1406, 274.7557) (292.253, 274.3017) (292.3676, 273.8487) (292.4843, 273.3966) (292.6033, 272.9455) (292.7246, 272.4953) (292.8481, 272.0461) (292.974, 271.598) (293.1023, 271.1509) (293.233, 270.705) (293.3661, 270.2601) (293.5018, 269.8165) (293.64, 269.3739) (293.7807, 268.9326) (293.924, 268.4924) (294.0699, 268.0535) (294.2186, 267.6159) (294.3701, 267.1797) (294.5246, 266.745) (294.6821, 266.3118) (294.8429, 265.8802) (295.0067, 265.4502) (295.1737, 265.0217) (295.3202, 264.6543) (295.4344, 264.3731) (295.515, 264.1775) (295.5609, 264.067) (295.5716, 264.0412) knots -1 -1 -1 -1 -1 -1 -0.98571429 -0.97142857 -0.95714286 -0.94285714 -0.92857143 -0.91428571 -0.9 -0.88571429 -0.87142857 -0.85714286 -0.84285714 -0.82857143 -0.81428571 -0.8 -0.78571429 -0.77142857 -0.75714286 -0.74285714 -0.72857143 -0.71428571 -0.7 -0.68571429 -0.67142857 -0.65714286 -0.64285714 -0.62857143 -0.61428571 -0.6 -0.58571429 -0.57142857 -0.55714286 -0.54285714 -0.52857143 -0.51428571 -0.5 -0.48571429 -0.47142857 -0.45714286 -0.44285714 -0.42857143 -0.41428571 -0.4 -0.38571429 -0.37142857 -0.35714286 -0.34285714 -0.32857143 -0.31428571 -0.3 -0.28571429 -0.27142857 -0.25714286 -0.24285714 -0.22857143 -0.21428571 -0.2 -0.18571429 -0.17142857 -0.15714286 -0.14285714 -0.13851185 -0.13851185 -0.13851185 -0.13851185 -0.13851185 -0.13851185
  spline S59 degree 3 poles (294.9688, 262.0993) (295.1423, 262.2117) (295.2922, 262.3569) (295.5279, 262.6966) (295.6114, 262.8878) (295.6909, 263.2479) (295.7014, 263.4105) (295.6727, 263.7333) (295.6338, 263.8916) (295.5716, 264.0412) knots 0 0 0 0 0.062015 0.062015 0.12403 0.12403 0.172638 0.172638 0.221247 0.221247 0.221247 0.221247
  arc A30 (294.9688, 262.0993) -> (288.1174, 257.5213) centre (452.3696, 19.1166) ccw
  spline S60 degree 3 poles (286.0927, 257.7076) (286.2387, 257.5612) (286.4119, 257.4448) (286.7931, 257.2848) (286.9975, 257.2428) (287.3662, 257.2399) (287.5275, 257.2634) (287.8373, 257.3584) (287.984, 257.4294) (288.1174, 257.5213) knots 0 0 0 0 0.062015 0.062015 0.12403 0.12403 0.172638 0.172638 0.221247 0.221247 0.221247 0.221247
  spline S61 degree 5 poles (286.0927, 257.7076) (286.073, 257.7274) (285.9884, 257.8121) (285.8385, 257.9613) (285.6225, 258.1745) (285.3391, 258.4504) (285.0071, 258.7687) (284.6726, 259.0846) (284.3353, 259.3983) (283.9954, 259.7096) (283.6529, 260.0187) (283.3079, 260.3256) (282.9605, 260.6304) (282.6108, 260.9332) (282.259, 261.234) (281.9051, 261.5329) (281.5491, 261.8299) (281.1911, 262.1251) (280.8311, 262.4183) (280.4691, 262.7097) (280.1052, 262.9993) (279.7393, 263.2871) (279.3716, 263.5731) (279.0021, 263.8574) (278.6309, 264.14) (278.2579, 264.4209) (277.8832, 264.7001) (277.5068, 264.9777) (277.1287, 265.2536) (276.749, 265.5279) (276.3677, 265.8005) (275.9848, 266.0716) (275.6003, 266.3411) (275.2143, 266.609) (274.8268, 266.8753) (274.4378, 267.1401) (274.0473, 267.4034) (273.6554, 267.6651) (273.262, 267.9253) (272.8672, 268.1841) (272.471, 268.4413) (272.0734, 268.697) (271.6744, 268.9513) (271.2741, 269.2041) (270.8724, 269.4555) (270.4695, 269.7054) (270.0652, 269.9538) (269.6596, 270.2009) (269.2527, 270.4465) (268.8446, 270.6907) (268.4352, 270.9335) (268.0246, 271.1748) (267.6128, 271.4148) (267.1997, 271.6534) (266.7854, 271.8906) (266.37, 272.1265) (265.9533, 272.3609) (265.5355, 272.594) (265.1166, 272.8258) (264.6965, 273.0561) (264.2753, 273.2852) (263.8529, 273.5129) (263.5141, 273.6939) (263.2595, 273.8292) (263.0896, 273.919) (263.0046, 273.9639) knots 0.13851185 0.13851185 0.13851185 0.13851185 0.13851185 0.13851185 0.14285714 0.15714286 0.17142857 0.18571429 0.2 0.21428571 0.22857143 0.24285714 0.25714286 0.27142857 0.28571429 0.3 0.31428571 0.32857143 0.34285714 0.35714286 0.37142857 0.38571429 0.4 0.41428571 0.42857143 0.44285714 0.45714286 0.47142857 0.48571429 0.5 0.51428571 0.52857143 0.54285714 0.55714286 0.57142857 0.58571429 0.6 0.61428571 0.62857143 0.64285714 0.65714286 0.67142857 0.68571429 0.7 0.71428571 0.72857143 0.74285714 0.75714286 0.77142857 0.78571429 0.8 0.81428571 0.82857143 0.84285714 0.85714286 0.87142857 0.88571429 0.9 0.91428571 0.92857143 0.94285714 0.95714286 0.97142857 0.98571429 1 1 1 1 1 1
  arc A31 (263.0046, 273.9639) -> (255.2172, 267.9885) centre (452.3696, 19.1166) ccw
  spline S62 degree 5 poles (255.2172, 267.9885) (255.2386, 267.8947) (255.2814, 267.7073) (255.3461, 267.4264) (255.4333, 267.0523) (255.5439, 266.5854) (255.6561, 266.1192) (255.7699, 265.6538) (255.8854, 265.1892) (256.0024, 264.7253) (256.121, 264.2622) (256.2413, 263.7998) (256.3632, 263.3383) (256.4867, 262.8775) (256.612, 262.4176) (256.7388, 261.9585) (256.8674, 261.5002) (256.9976, 261.0428) (257.1296, 260.5863) (257.2632, 260.1306) (257.3986, 259.6757) (257.5357, 259.2218) (257.6745, 258.7688) (257.8151, 258.3167) (257.9574, 257.8655) (258.1016, 257.4153) (258.2475, 256.966) (258.3952, 256.5177) (258.5447, 256.0703) (258.6961, 255.624) (258.8493, 255.1787) (259.0044, 254.7344) (259.1614, 254.2911) (259.3203, 253.8489) (259.4811, 253.4078) (259.6438, 252.9678) (259.8085, 252.5289) (259.9751, 252.0912) (260.1438, 251.6546) (260.3145, 251.2192) (260.4872, 250.785) (260.662, 250.352) (260.8388, 249.9202) (261.0178, 249.4897) (261.1989, 249.0606) (261.3822, 248.6327) (261.5678, 248.2062) (261.7555, 247.7811) (261.9456, 247.3575) (262.138, 246.9353) (262.3328, 246.5146) (262.5299, 246.0953) (262.7294, 245.6777) (262.9314, 245.2616) (263.1359, 244.8471) (263.343, 244.4344) (263.553, 244.0236) (263.7657, 243.6147) (263.9814, 243.2077) (264.2, 242.8028) (264.4215, 242.3998) (264.6147, 242.0546) (264.7646, 241.7908) (264.87, 241.6074) (264.9299, 241.5037) (264.9439, 241.4796) knots -1 -1 -1 -1 -1 -1 -0.98571429 -0.97142857 -0.95714286 -0.94285714 -0.92857143 -0.91428571 -0.9 -0.88571429 -0.87142857 -0.85714286 -0.84285714 -0.82857143 -0.81428571 -0.8 -0.78571429 -0.77142857 -0.75714286 -0.74285714 -0.72857143 -0.71428571 -0.7 -0.68571429 -0.67142857 -0.65714286 -0.64285714 -0.62857143 -0.61428571 -0.6 -0.58571429 -0.57142857 -0.55714286 -0.54285714 -0.52857143 -0.51428571 -0.5 -0.48571429 -0.47142857 -0.45714286 -0.44285714 -0.42857143 -0.41428571 -0.4 -0.38571429 -0.37142857 -0.35714286 -0.34285714 -0.32857143 -0.31428571 -0.3 -0.28571429 -0.27142857 -0.25714286 -0.24285714 -0.22857143 -0.21428571 -0.2 -0.18571429 -0.17142857 -0.15714286 -0.14285714 -0.13851185 -0.13851185 -0.13851185 -0.13851185 -0.13851185 -0.13851185
  spline S63 degree 3 poles (264.5998, 239.4756) (264.7572, 239.6097) (264.8868, 239.7732) (265.0761, 240.1408) (265.134, 240.3413) (265.1658, 240.7086) (265.1549, 240.8712) (265.0844, 241.1875) (265.0251, 241.3394) (264.9439, 241.4796) knots 0 0 0 0 0.062015 0.062015 0.12403 0.12403 0.172638 0.172638 0.221247 0.221247 0.221247 0.221247
  arc A32 (264.5998, 239.4756) -> (258.4046, 234.0425) centre (452.3696, 19.1166) ccw
  spline S64 degree 3 poles (256.3729, 233.9629) (256.5367, 233.8369) (256.7236, 233.744) (257.1224, 233.6352) (257.3306, 233.6202) (257.6965, 233.6654) (257.8533, 233.7098) (258.1481, 233.8445) (258.2843, 233.934) (258.4046, 234.0425) knots 0 0 0 0 0.062015 0.062015 0.12403 0.12403 0.172638 0.172638 0.221247 0.221247 0.221247 0.221247
  spline S65 degree 5 poles (256.3729, 233.9629) (256.3507, 233.98) (256.2558, 234.0529) (256.0877, 234.1813) (255.8457, 234.3644) (255.5287, 234.601) (255.1581, 234.8732) (254.7851, 235.1428) (254.4098, 235.4098) (254.0322, 235.6741) (253.6522, 235.9358) (253.2701, 236.1951) (252.8859, 236.4519) (252.4997, 236.7065) (252.1117, 236.9588) (251.7218, 237.209) (251.3301, 237.457) (250.9366, 237.7028) (250.5414, 237.9466) (250.1445, 238.1882) (249.7458, 238.4278) (249.3456, 238.6654) (248.9437, 238.901) (248.5402, 239.1347) (248.1353, 239.3664) (247.7288, 239.5962) (247.3208, 239.8241) (246.9114, 240.0501) (246.5006, 240.2743) (246.0883, 240.4967) (245.6747, 240.7173) (245.2597, 240.936) (244.8433, 241.153) (244.4257, 241.3682) (244.0067, 241.5817) (243.5865, 241.7935) (243.165, 242.0035) (242.7422, 242.2119) (242.3182, 242.4185) (241.893, 242.6235) (241.4666, 242.8268) (241.039, 243.0285) (240.6103, 243.2285) (240.1804, 243.4269) (239.7494, 243.6237) (239.3172, 243.8188) (238.884, 244.0124) (238.4496, 244.2044) (238.0142, 244.3948) (237.5777, 244.5836) (237.1401, 244.7709) (236.7015, 244.9566) (236.2619, 245.1408) (235.8212, 245.3234) (235.3795, 245.5045) (234.9368, 245.6841) (234.4931, 245.8622) (234.0485, 246.0388) (233.6029, 246.2138) (233.1563, 246.3874) (232.7088, 246.5595) (232.2603, 246.7301) (231.9008, 246.8654) (231.6307, 246.9662) (231.4505, 247.0332) (231.3604, 247.0665) knots 0.13851185 0.13851185 0.13851185 0.13851185 0.13851185 0.13851185 0.14285714 0.15714286 0.17142857 0.18571429 0.2 0.21428571 0.22857143 0.24285714 0.25714286 0.27142857 0.28571429 0.3 0.31428571 0.32857143 0.34285714 0.35714286 0.37142857 0.38571429 0.4 0.41428571 0.42857143 0.44285714 0.45714286 0.47142857 0.48571429 0.5 0.51428571 0.52857143 0.54285714 0.55714286 0.57142857 0.58571429 0.6 0.61428571 0.62857143 0.64285714 0.65714286 0.67142857 0.68571429 0.7 0.71428571 0.72857143 0.74285714 0.75714286 0.77142857 0.78571429 0.8 0.81428571 0.82857143 0.84285714 0.85714286 0.87142857 0.88571429 0.9 0.91428571 0.92857143 0.94285714 0.95714286 0.97142857 0.98571429 1 1 1 1 1 1
  arc A33 (231.3604, 247.0665) -> (224.4196, 240.1258) centre (452.3696, 19.1166) ccw